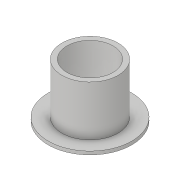
# Autodesk Inventor part: espaciador
Saved by Autodesk Inventor 2019 (Build 230136000, 136)
## iProperties
Created: 2019-11-14
Part Number: espaciador
Material: Generic
Document SubType Name: Modeling
Designer: Carlos Andres garcia velez
Density: 1 g/cm^3
Appearance: Default
Author: Carlos Andres garcia velez
## iProperties of the stored document espaciador_3DPrint.ipt
Created: 2019-11-14
Part Number: espaciador_3DPrint
Material: Generic
Document SubType Name: Modeling
Designer: Carlos Andres garcia velez
Density: 1 g/cm^3
Appearance: Default
Author: Carlos Andres garcia velez
Autodesk Inventor part; units mm, degrees
ref_plane "YZ Plane" through (0, 0, 0) normal (1, 0, 0) x (0, 1, 0)
ref_plane "XZ Plane" through (0, 0, 0) normal (0, 1, 0) x (-1, 0, 0)
ref_plane "XY Plane" through (0, 0, 0) normal (0, 0, 1) x (1, 0, 0)
sketch "Sketch1" plane through (0, 0, 0) normal (1, 0, 0) x (0, 1, 0)
  line L0 (7.8554, 0) -> (-4.9831, 0) construction
  line L1 (8.8316, -6.9) -> (-7.1684, -6.9)
  line L2 (-7.1684, -6.9) -> (-7.1684, -12.5)
  line L3 (-7.1684, -12.5) -> (-6.1684, -12.5)
  line L4 (-6.1684, -12.5) -> (-6.1684, -8.4)
  line L5 (-6.1684, -8.4) -> (8.8316, -8.4)
  line L6 (8.8316, -6.9) -> (8.8316, -8.4)
  point P0 (0, 0)
  dimension "d0" = 6.9
  dimension "d1" = 8.4
  dimension "d2" = 12.5
  dimension "d3" = 0
  dimension "d4" = 16
  dimension "d5" = 1
  constraints: 14 end point, 5 perpendicular, 2 horizontal
  measures "d0" distance between parallel lines of L0 L1
  measures "d1" distance between parallel lines of L0 L5
  measures "d2" distance between parallel lines of L0 L3
  measures "d3" distance from line of point (0, 0) L0
  measures "d4" distance of L1.start L1.end
  measures "d5" distance of L2.end L3.end
revolve "Revolution1" add sketch "Sketch1" angle 360 about axis through (0, 7.8554, 0) along (0, -1, 0)
body "Solid1"
